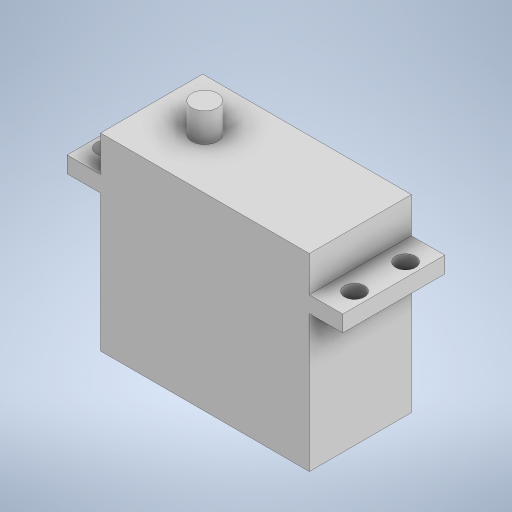
# Autodesk Inventor part: servo
Saved by Autodesk Inventor 2024.3 (Build 283343000, 343)
## iProperties
Created: 2024-10-22
Part Number: servo
Material: 一般
Document SubType Name: Modeling
Designer: 佐藤智貴
Density: 1 g/cm^3
Appearance: 既定
Project: MG996R
Author: 佐藤智貴
Title: MG996R
Autodesk Inventor part; units mm, degrees
ref_plane "YZ Plane" through (0, 0, 0) normal (1, 0, 0) x (0, 1, 0)
ref_plane "XZ Plane" through (0, 0, 0) normal (0, 1, 0) x (-1, 0, 0)
ref_plane "XY Plane" through (0, 0, 0) normal (0, 0, 1) x (1, 0, 0)
sketch "スケッチ12" plane through (0, 0, 0) normal (0, 0, 1) x (1, 0, 0)
  line L0 (0, 0) -> (54, 0)
  line L1 (54, 0) -> (54, 37)
  line L2 (54, 37) -> (0, 37)
  line L3 (0, 37) -> (0, 0)
  dimension "d76" = 54
  dimension "d77" = 37
  constraints: 8 end point, 2 parallel, 1 horizontal, 1 perpendicular
  measures "d76" distance of L1.end L2.end
  measures "d77" distance of L0.end L1.end
extrude "押し出し7" add sketch "スケッチ12" along normal blind 20
sketch "スケッチ14" plane through (0, 37, 0) normal (0, 1, 0) x (1, 0, 0)
  line L0 (54, 0) -> (54, -20) projected
  line L1 (54, 0) -> (0, 0) projected
  line L2 (0, 0) -> (0, -20) projected
  point P0 (2.7, -5)
  point P1 (2.7, -15)
  point P2 (51.3, -5)
  point P3 (51.3, -15)
  dimension "d80" = 48.6
  dimension "d81" = 10
  dimension "d82" = 10
  dimension "d83" = 2.7
  dimension "d84" = 5
  dimension "d85" = 5
  dimension "d86" = 2.7
  dimension "d87" = 2.7
  measures "d80" distance of point (51.3, -5) point (2.7, -5)
  measures "d81" distance of point (2.7, -15) point (2.7, -5)
  measures "d82" distance of point (51.3, -15) point (51.3, -5)
  measures "d83" distance from line of L0 point (51.3, -5)
  measures "d84" distance from line of L1 point (51.3, -5)
  measures "d85" distance from line of L1 point (2.7, -5)
  measures "d86" distance from line of L2 point (2.7, -15)
  measures "d87" distance from line of L0 point (51.3, -15)
hole "穴3" at (2.7, 37, 5) at (2.7, 37, 15) at (51.3, 37, 5) at (51.3, 37, 15) direction (0, -1, 0) diameter 3.9 end through all
sketch "スケッチ15" plane through (0, 0, 20) normal (0, 0, 1) x (1, 0, 0)
  line L0 (0, 0) -> (6.55, 0)
  line L1 (6.55, 0) -> (6.55, 26.8)
  line L2 (6.55, 26.8) -> (0, 26.8)
  line L3 (0, 26.8) -> (0, 0)
  line L4 (54, 0) -> (54, 37) projected
  line L5 (54, 0) -> (47.45, 0)
  line L6 (47.45, 0) -> (47.45, 26.8)
  line L7 (47.45, 26.8) -> (54, 26.8)
  line L8 (54, 26.8) -> (54, 0)
  line L9 (54, 37) -> (0, 37) projected
  line L10 (0, 37) -> (6.55, 37)
  line L11 (6.55, 37) -> (6.55, 30)
  line L12 (6.55, 30) -> (0, 30)
  line L13 (0, 30) -> (0, 37)
  line L14 (54, 37) -> (47.45, 37)
  line L15 (47.45, 37) -> (47.45, 30)
  line L16 (47.45, 30) -> (54, 30)
  line L17 (54, 30) -> (54, 37)
  dimension "d100" = 26.8
  dimension "d101" = 6.55
  dimension "d102" = 40.9
  dimension "d103" = 7
  constraints: 32 end point, 8 parallel, 4 horizontal, 4 perpendicular, 2 point on line
  measures "d100" distance of L0.end L1.end
  measures "d101" distance between parallel lines of L3 L1
  measures "d102" distance between parallel lines of L6 L1
  measures "d103" distance of L10.end L11.end
extrude "押し出し8" cut sketch "スケッチ15" against normal blind 20
sketch "スケッチ16" plane through (6.55, 37, 0) normal (0, 1, 0) x (1, 0, 0)
  line L0 (47.45, -20) -> (47.45, 0) projected
  line L1 (47.45, -10) -> (-12.7368, -10)
  line L2 (-6.55, -20) -> (-6.55, 0) projected
  circle A0 centre (10.4, -10) radius 2.5
  circle A1 centre (44.75, -15) radius 1.95 projected
  dimension "d106" = 5
  dimension "d107" = 34.35
  constraints: 2 end point, 1 centre point, 1 midpoint, 1 perpendicular, 1 point on line
  measures "d106" diameter of A0
  measures "d107" horizontal distance of A0.centre A1.centre
extrude "押し出し9" add sketch "スケッチ16" along normal blind 5.7 contours A0 L1 | L1 A0
equation "\"d85\" = d84"
equation "\"d86\" = d83"
